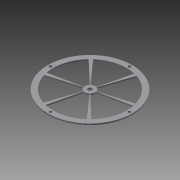
# Autodesk Inventor part: Flywheel Hub
Saved by Autodesk Inventor 2013 (Build 170138000, 138)
## iProperties
Created: 2013-01-17
Part Number: Flywheel Hub
Material: Generic
Document SubType Name: Modeling
Designer: actoennies
Density: 1 g/cm^3
Mass: 31.4711 g
Surface Area: 269.866 cm^2
Volume: 31.4711 cm^3
Author: actoennies
Autodesk Inventor part; units mm, degrees
ref_plane "YZ Plane" through (0, 0, 0) normal (1, 0, 0) x (0, 1, 0)
ref_plane "XZ Plane" through (0, 0, 0) normal (0, 1, 0) x (-1, 0, 0)
ref_plane "XY Plane" through (0, 0, 0) normal (0, 0, 1) x (1, 0, 0)
sketch "Sketch1" plane through (0, 0, 0) normal (0, 1, 0) x (-1, 0, 0)
  circle A0 centre (0, 0) radius 101.6
  circle A1 centre (0, 95.25) radius 3.3782
  circle A2 centre (-95.25, 0) radius 3.3782
  circle A3 centre (95.25, 0) radius 3.3782
  circle A4 centre (0, -95.25) radius 3.3782
  circle A5 centre (0, 0) radius 95.25 construction
  line L0 (2.7496, 4.7625) -> (5.4993, 0)
  line L1 (5.4993, 0) -> (2.7496, -4.7625)
  line L2 (2.7496, -4.7625) -> (-2.7496, -4.7625)
  line L3 (-2.7496, -4.7625) -> (-5.4993, 0)
  line L4 (-5.4993, 0) -> (-2.7496, 4.7625)
  line L5 (-2.7496, 4.7625) -> (2.7496, 4.7625)
  line L6 (-4.0354, -12.0418) -> (-28.2478, -84.2928)
  line L7 (-2.9705, -12.3477) -> (-20.7937, -86.434)
  line L8 (8.4108, -9.5157) -> (58.8758, -66.6097)
  line L9 (9.2082, -8.7464) -> (64.4572, -61.2248)
  line L10 (12.4462, 2.5262) -> (87.1236, 17.6831)
  line L11 (12.1787, 3.6013) -> (85.2509, 25.2091)
  line L12 (4.0354, 12.0418) -> (28.2478, 84.2928)
  line L13 (2.9705, 12.3477) -> (20.7937, 86.434)
  line L14 (-8.4108, 9.5157) -> (-58.8758, 66.6097)
  line L15 (-9.2082, 8.7464) -> (-64.4572, 61.2248)
  line L16 (-12.4462, -2.5262) -> (-87.1236, -17.6831)
  line L17 (-12.1787, -3.6013) -> (-85.2509, -25.2091)
  arc A6 (2.9705, 12.3477) -> (-8.4108, 9.5157) centre (0, 0) ccw
  arc A7 (12.1787, 3.6013) -> (4.0354, 12.0418) centre (0, 0) ccw
  arc A8 (9.2082, -8.7464) -> (12.4462, 2.5262) centre (0, 0) ccw
  arc A9 (-2.9705, -12.3477) -> (8.4108, -9.5157) centre (0, 0) ccw
  arc A10 (-9.2082, 8.7464) -> (-12.4462, -2.5262) centre (0, 0) ccw
  arc A11 (-12.1787, -3.6013) -> (-4.0354, -12.0418) centre (0, 0) ccw
  arc A12 (-85.2509, -25.2091) -> (-28.2478, -84.2928) centre (0, 0) ccw
  arc A13 (-64.4572, 61.2248) -> (-87.1236, -17.6831) centre (0, 0) ccw
  arc A14 (20.7937, 86.434) -> (-58.8758, 66.6097) centre (0, 0) ccw
  arc A15 (85.2509, 25.2091) -> (28.2478, 84.2928) centre (0, 0) ccw
  arc A16 (-20.7937, -86.434) -> (58.8758, -66.6097) centre (0, 0) ccw
  arc A17 (64.4572, -61.2248) -> (87.1236, 17.6831) centre (0, 0) ccw
  dimension "d0" = 203.2
  dimension "d2" = 6.7564
  dimension "d3" = 6.7564
  dimension "d4" = 6.7564
  dimension "d5" = 6.7564
  dimension "d6" = 190.5
  dimension "d7" = 95.25
  dimension "d8" = 95.25
  dimension "d9" = 95.25
  dimension "d10" = 95.25
  dimension "d13" = 9.525
  dimension "d14" = 0
  dimension "d15" = 0
  dimension "d16" = 5
  dimension "d19" = 360
  constraints: 36 end point, 24 point on circle, 18 centre point, 5 coincident, 50 other
  measures "d0" diameter of A0
  measures "d2" diameter of A1
  measures "d3" diameter of A2
  measures "d4" diameter of A3
  measures "d5" diameter of A4
  measures "d6" diameter of A5
  measures "d7" distance of A5.centre A1.centre
  measures "d8" distance of point (0, 0) A2.centre
  measures "d9" distance of A3.centre point (0, 0)
  measures "d10" distance of point (0, 0) A4.centre
  measures "d13" distance between parallel lines of L5 L2
  measures "d14" distance from line of point (0, 0) L6
  measures "d15" distance from line of point (0, 0) L7
  measures "d16" angle of L6 L7
extrude "Extrusion1" add sketch "Sketch1" along normal blind 3.175
body "Solid1"
